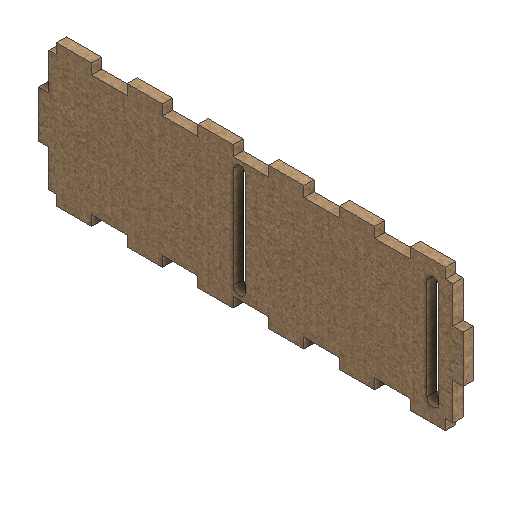
# Autodesk Inventor part: FloorPlate
Saved by Autodesk Inventor 2025.2 (Build 292293000, 293)
## iProperties
Created: 2025-03-07
Part Number: FloorPlate
Material: MDF Medium Density Fiberboard
Document SubType Name: Modeling
Designer: ahorat
Density: 0.8 g/cm^3
Appearance: Cardboard - Corrugated
Author: ahorat
Autodesk Inventor part; units mm, degrees
ref_plane "YZ Plane" through (0, 0, 0) normal (1, 0, 0) x (0, 1, 0)
ref_plane "XZ Plane" through (0, 0, 0) normal (0, 1, 0) x (-1, 0, 0)
ref_plane "XY Plane" through (0, 0, 0) normal (0, 0, 1) x (1, 0, 0)
sketch "Sketch1" plane through (0, 0, 0) normal (0, 0, 1) x (1, 0, 0)
  line L0 (-105, -35) -> (105, -35)
  line L1 (105, -35) -> (105, 35)
  line L2 (105, 35) -> (-105, 35)
  line L3 (-105, 35) -> (-105, -35)
  line L4 (-105, -35) -> (105, 35) construction
  line L5 (105, -35) -> (-105, 35) construction
  point P0 (0, 0)
  dimension "d0" = 210
  dimension "d1" = 70
  constraints: 12 end point, 2 midpoint, 2 parallel, 1 horizontal, 1 perpendicular
  measures "d0" distance of L1.end L2.end
  measures "d1" distance of L0.end L1.end
extrude "Extrusion1" add sketch "Sketch1" along normal blind 5
sketch "Sketch2" plane through (0, 0, 5) normal (0, 0, 1) x (1, 0, 0)
  line L0 (105, 35) -> (-105, 35) projected
  line L1 (-8.8, 35) -> (-8.8, 29.9)
  line L2 (-8.8, 29.9) -> (8.8, 29.9)
  line L3 (8.8, 29.9) -> (8.8, 35)
  line L4 (-43.8, 35) -> (-43.8, 29.9)
  line L5 (-43.8, 29.9) -> (-26.2, 29.9)
  line L6 (-26.2, 29.9) -> (-26.2, 35)
  line L7 (-78.8, 35) -> (-78.8, 29.9)
  line L8 (-78.8, 29.9) -> (-61.2, 29.9)
  line L9 (-61.2, 29.9) -> (-61.2, 35)
  line L10 (-113.8, 35) -> (-113.8, 29.9)
  line L11 (-113.8, 29.9) -> (-96.2, 29.9)
  line L12 (-96.2, 29.9) -> (-96.2, 35)
  line L13 (43.8, 29.9) -> (43.8, 35)
  line L14 (26.2, 29.9) -> (43.8, 29.9)
  line L15 (26.2, 35) -> (26.2, 29.9)
  line L16 (78.8, 29.9) -> (78.8, 35)
  line L17 (61.2, 29.9) -> (78.8, 29.9)
  line L18 (61.2, 35) -> (61.2, 29.9)
  line L19 (113.8, 29.9) -> (113.8, 35)
  line L20 (96.2, 29.9) -> (113.8, 29.9)
  line L21 (96.2, 35) -> (96.2, 29.9)
  line L22 (105, -35) -> (105, 35) projected
  line L23 (105, 35) -> (-105, 35) projected
  line L24 (-105, 35) -> (-105, -35) projected
  line L25 (-105, -35) -> (105, -35) projected
  line L26 (-99.9, 29.9) -> (-99.9, 11.6167)
  line L27 (-99.9, 11.6167) -> (-105, 11.6167)
  line L28 (99.9, 29.9) -> (99.9, 11.6167)
  line L29 (99.9, 11.6167) -> (105, 11.6167)
  point P0 (0, 0)
  point P1 (0, 35)
  point P2 (0, 29.9)
  point P3 (-8.8, 32.45)
  point P4 (8.8, 32.45)
  point P5 (-43.8, 32.45)
  point P6 (-35, 29.9)
  point P7 (-26.2, 32.45)
  point P8 (-35, 35)
  point P9 (-78.8, 32.45)
  point P10 (-70, 29.9)
  point P11 (-61.2, 32.45)
  point P12 (-70, 35)
  point P13 (-113.8, 32.45)
  point P14 (-105, 29.9)
  point P15 (-96.2, 32.45)
  point P16 (-105, 35)
  point P17 (26.2, 32.45)
  point P18 (35, 35)
  point P19 (35, 29.9)
  point P20 (43.8, 32.45)
  point P21 (61.2, 32.45)
  point P22 (70, 35)
  point P23 (70, 29.9)
  point P24 (78.8, 32.45)
  point P25 (96.2, 32.45)
  point P26 (105, 35)
  point P27 (105, 29.9)
  point P28 (113.8, 32.45)
  point P29 (105, 29.9)
  point P30 (-105, 35)
  point P31 (-105, 29.9)
  point P32 (-102.45, 11.6167)
  dimension "d4" = 5.1
  dimension "d5" = 17.6
  dimension "d6" = 210
  dimension "d24" = 35
  dimension "d31" = 35
  dimension "d36" = 70
  dimension "d37" = 23.3833
  constraints: 50 end point, 8 point on line, 6 perpendicular, 5 midpoint, 2 horizontal, 2 vertical, 1 vertical alignment, 66 other
  measures "d4" distance between parallel lines of L0 L2
  measures "d5" distance of point (-8.8, 32.45) point (8.8, 32.45)
  measures "d6" distance of L0.start L0.end
  measures "d24" distance of L1.start L4.start
  measures "d31" distance of point (-8.8, 32.45) point (26.2, 32.45)
  measures "d36" distance of L23.end L24.end
  measures "d37" distance from line of L0 point (-102.45, 11.617)
extrude "Extrusion2" cut sketch "Sketch2" against normal blind 5 contours L22 L20 L21 L0 | L22 L29 L28 L20 | L16 L17 L18 L0 | L13 L14 L15 L0 | L24 L11 L26 L27 | L3 L2 L1 L0 | L24 L0 L12 L11 | L6 L5 L4 L0 | L0 L9 L8 L7
sketch "Sketch4" plane through (0, 0, 0) normal (0, 0, -1) x (-1, 0, 0)
  line L0 (-85, -26.99) -> (0.6, -26.99)
  line L1 (0.6, -26.99) -> (0.6, 26.99)
  line L2 (0.6, 26.99) -> (-85, 26.99)
  line L3 (-85, 26.99) -> (-85, -26.99)
  line L4 (-85, -26.99) -> (0.6, 26.99) construction
  line L5 (0.6, -26.99) -> (-85, 26.99) construction
  line L6 (-105, -35) -> (-105, 35) projected
  line L7 (-85, 26.99) -> (0.0055, 26.99) construction
  line L8 (0.0055, 26.99) -> (0.0055, -27.0274) construction
  line L9 (0.0055, -27.0274) -> (-85, -27.0274) construction
  line L10 (-85, -27.0274) -> (-85, 26.99) construction
  point P0 (0, 0)
  point P1 (-42.2, 0)
  point P2 (-105, 29.9)
  dimension "d16" = 53.98
  dimension "d17" = 85.6
  dimension "d18" = 20
  constraints: 12 end point, 2 midpoint, 2 parallel, 1 horizontal, 1 horizontal alignment, 1 perpendicular, 2 other
  measures "d16" distance of L0.end L1.end
  measures "d17" distance of L1.end L2.end
  measures "d18" distance between parallel lines of L6 L3
extrude "Extrusion4" cut sketch "Sketch4" against normal blind 0.5
sketch "Sketch3" plane through (0, 0, 0) normal (0, 0, -1) x (-1, 0, 0)
  line L0 (8.6, 25) -> (2.6, 25) construction
  line L1 (2.6, 25) -> (2.6, -25)
  line L2 (2.6, -25) -> (8.6, -25) construction
  line L3 (8.6, -25) -> (8.6, 25)
  line L4 (8.6, 25) -> (2.6, -25) construction
  line L5 (2.6, 25) -> (8.6, -25) construction
  arc A0 (2.6, -25) -> (8.6, -25) centre (5.6, -25) ccw
  arc A1 (8.6, 25) -> (2.6, 25) centre (5.6, 25) ccw
  line L6 (0.6, 26.99) -> (0.6, -26.99) projected
  line L7 (-85, 26.99) -> (0.6, 26.99) projected
  line L8 (-42.2, 26.99) -> (-42.2, -26.99)
  line L9 (0.6, -26.99) -> (-85, -26.99) projected
  line L10 (-93, 25) -> (-87, 25) construction
  line L11 (-87, 25) -> (-87, -25)
  line L12 (-87, -25) -> (-93, -25) construction
  line L13 (-93, -25) -> (-93, 25)
  line L14 (-93, 25) -> (-87, -25) construction
  line L15 (-87, 25) -> (-93, -25) construction
  arc A2 (-93, -25) -> (-87, -25) centre (-90, -25) ccw
  arc A3 (-87, 25) -> (-93, 25) centre (-90, 25) ccw
  point P0 (0, 0)
  point P1 (5.6, 0)
  point P2 (-90, 0)
  dimension "d12" = 6
  dimension "d13" = 50
  dimension "d21" = 5
  constraints: 26 end point, 8 point on circle, 7 symmetric about line, 4 centre point, 4 midpoint, 2 parallel, 2 tangent, 1 horizontal, 1 horizontal alignment, 1 perpendicular, 2 other
  measures "d12" distance between parallel lines of L3 L1
  measures "d13" distance of L0.end L1.end
  measures "d21" distance from line of L6 point (5.6, 0)
extrude "Extrusion3" cut sketch "Sketch3" against normal blind 5 contours A1 L3 A0 L1 | L11 A2 L13 A3
mirror "Mirror2" about plane through (0, 0, 0) normal (0, 1, 0) of "Extrusion2"
sketch "Sketch5" plane through (0, 0, 0.5) normal (0, 0, -1) x (-1, 0, 0)
  line L0 (-85, 26.99) -> (0.0055, 26.99) construction
  line L1 (0.0055, 26.99) -> (0.0055, -27.0274) construction
  line L2 (0.0055, -27.0274) -> (-85, -27.0274) construction
  line L3 (-85, -27.0274) -> (-85, 26.99) construction
  point P0 (0, 0)
  constraints: 2 other
equation "\"d24\" = 0.166667 * d6"
equation "\"d31\" = 0.166667 * d6"
body "Solid1"
